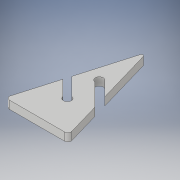
# Autodesk Inventor part: directional_arrow
Saved by Autodesk Inventor 2019 (Build 230136000, 136)
## iProperties
Created: 2019-04-03
Part Number: directional_arrow
Material: Generic
Document SubType Name: Modeling
Designer: jmc
Density: 1 g/cm^3
Appearance: Default
Author: jmc
URL: https://www.amazon.es/MagiDeal-Marcador-Flecha-Triangular-Naufragios/dp/B07CHZN8H6
Autodesk Inventor part; units mm, degrees
ref_plane "YZ Plane" through (0, 0, 0) normal (1, 0, 0) x (0, 1, 0)
ref_plane "XZ Plane" through (0, 0, 0) normal (0, 1, 0) x (-1, 0, 0)
ref_plane "XY Plane" through (0, 0, 0) normal (0, 0, 1) x (1, 0, 0)
sketch "Sketch1" plane through (0, 0, 0) normal (0, 1, 0) x (-1, 0, 0)
  line L0 (0, 0) -> (0, -40) construction
  line L1 (0, -40) -> (0, 29.0613) construction
  line L2 (0, 29.0613) -> (17.3386, 29.0613)
  line L3 (0, 29.0613) -> (-17.3386, 29.0613)
  arc A0 (19.2597, 26.505) -> (17.3386, 29.0613) centre (17.3386, 27.0613) ccw
  arc A1 (-17.3386, 29.0613) -> (-19.2597, 26.505) centre (-17.3386, 27.0613) ccw
  arc A2 (-0.9605, -36.6832) -> (0.9605, -36.6832) centre (0, -36.4051) ccw
  line L4 (0, 0) -> (0, 10) construction
  line L5 (0, 10) -> (0, -10) construction
  arc A3 (2.4749, 10.3536) -> (0, 7.5) centre (0, 10) ccw
  arc A4 (-1.7678, -11.7678) -> (0, -7.5) centre (0, -10) ccw
  line L6 (2.4749, 10.3536) -> (11.8634, 0.965)
  line L7 (-0.3536, 7.5251) -> (10.5931, -3.4215)
  line L8 (-1.7678, -11.7678) -> (-10.7883, -2.7472)
  line L9 (0.3536, -7.5251) -> (-13.3826, 6.211)
  line L10 (19.2597, 26.505) -> (11.8634, 0.965)
  line L11 (10.5931, -3.4215) -> (0.9605, -36.6832)
  line L12 (-19.2597, 26.505) -> (-13.3826, 6.211)
  line L13 (-10.7883, -2.7472) -> (-0.9605, -36.6832)
  point P0 (20, 29.0613)
  point P1 (-20, 29.0613)
  dimension "d0" = 40
  dimension "d1" = 20
  dimension "d2" = 20
  dimension "d3" = 2
  dimension "d4" = 2
  dimension "d5" = 1
  dimension "d6" = 10
  dimension "d7" = 20
  dimension "d8" = 5
  dimension "d9" = 5
  constraints: 28 end point, 12 point on circle, 10 tangent, 7 point on line, 5 centre point, 2 coincident, 2 horizontal, 1 parallel, 1 vertical
  measures "d0" distance of L0.start L0.end
  measures "d1" distance of L1.end point (20, 29.061)
  measures "d2" distance of L1.end point (-20, 29.061)
  measures "d3" radius of A0
  measures "d4" radius of A1
  measures "d5" radius of A2
  measures "d6" distance of L0.start L4.end
  measures "d7" distance of L4.end L5.end
  measures "d8" diameter of A3
  measures "d9" diameter of A4
extrude "Extrusion1" add sketch "Sketch1" along normal blind 5
body "Solid1"
